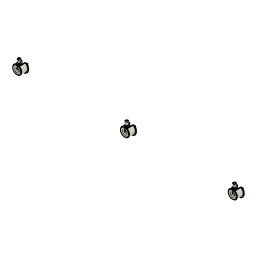
Rafix D20 Set (Autodesk Fusion 360 design; units mm, degrees)
description: Smart Rafix 20 Set
part number: Rafix 20 Set
description: Hafele Rafix S20 Connecting bolt
part number: Rafix S20 Bolt (263.20.xxx)
description: Hafele Rafix 20 Connector housing
part number: Rafix 20 (263.10.xxx)
Autodesk Fusion 360 part; units mm, degrees
sketch "Main Sketch" plane through (0, 0, 0) normal (0, 0, 1) x (1, 0, 0)
  line L0 (300, -10) -> (-300, -10)
  line L1 (-300, -10) -> (-300, 10)
  line L2 (-300, 10) -> (300, 10)
  line L3 (300, 10) -> (300, -10)
  line L4 (300, -10) -> (-300, 10) construction
  line L5 (-300, -10) -> (300, 10) construction
  circle A0 centre (-240, 0.5) radius 0.5
  circle A1 centre (240, 0.5) radius 0.5
  point P0 (-240, 0.5)
  point P1 (240, 0.5)
  dimension "d3" = 600
  dimension "d4" = 20
  dimension "d7" = 60
  dimension "d9" = 9.5
  dimension "d16" = 1
  dimension "d17" = 1
  dimension "d31" = 60
  constraint horizontal L0
  constraint perpendicular L0 L1
  constraint parallel L0 L2
  constraint parallel L1 L3
  constraint coincident L4 origin
  constraint coincident L5 origin
  constraint horizontal P0 P1
  constraint coincident P0 A0.centre
  constraint coincident P1 A1.centre
  measures "d3" distance of L0.start L0.end
  measures "d4" distance of L0 L2
  measures "d7" distance of L1 P0
  measures "d9" distance of L2 P0
  measures "d16" diameter of A0
  measures "d17" diameter of A1
  measures "d31" distance of L3 P1
extrude "Extrude3" add sketch "Main Sketch" along normal blind 10 contours A0 makes body 1
pattern_linear "R-Pattern1" count 3 spacing 240 along (1, 0, 0) of bodies 1 makes body 2 at (0.4994, 0.4751, 6.6667) makes body 3 at (240.0622, 0.0039, 3.3333)
ref_plane "WorkPlane1" through (-240, 0.5, 5) normal (-1, 0, 0) x (0, 0, 1)
sketch "Sketch2" plane through (-240, 0.5, 5) normal (-1, 0, 0) x (0, 1, 0)
  line L0 (0, 5) -> (0, -19.5056)
  line L1 (-1.5, 5) -> (-1.5, 3.5)
  line L2 (-1.5, 3.5) -> (-3, 3.5)
  line L3 (-3, 3.5) -> (-3, -6)
  line L4 (-10.5, 5) -> (9.5, 5)
  line L5 (-3, -6) -> (0, -6)
  line L6 (-1.5, 5) -> (-3.5, 5)
  line L7 (-3.5, 5) -> (-3.5, 8.5)
  line L8 (-3.5, 8.5) -> (-1.5, 8.5)
  line L9 (-1.5, 8.5) -> (-1.5, 11)
  line L10 (0, 14) -> (-3.5, 14)
  line L11 (-3.5, 14) -> (-3.5, 13.6)
  arc A0 (-3.5, 13.6) -> (-1.5, 11) centre (-0.81, 13.6) ccw
  line L12 (0, 5) -> (0, 14)
  point P0 (0, 5)
  point P1 (0, 5)
  dimension "d34" = 1.5
  dimension "d35" = 3
  dimension "d36" = 6
  dimension "d37" = 11
  dimension "d38" = 7
  dimension "d39" = 3.5
  dimension "d40" = 2.5
  dimension "d41" = 3
  dimension "d42" = 0.4
  dimension "d43" = 9
  dimension "d44" = 7
  constraint vertical L0
  constraint parallel L0 L1
  constraint perpendicular L1 L2
  constraint perpendicular L2 L3
  constraint coincident L1.start L4
  constraint coincident L0 L5.end
  constraint perpendicular L0 L5
  constraint coincident L4 L6.end
  constraint perpendicular L4 L7
  constraint perpendicular L1 L8
  constraint perpendicular L4 L9
  constraint horizontal L10
  constraint perpendicular L10 L11
  constraint coincident P0 L0.start
  constraint vertical L10.start P1
  constraint tangent L11 A0
  constraint coincident P1 P0
  measures "d34" distance of L2 L4
  measures "d37" distance of L3.end L4
  measures "d39" distance of L4 L8
  measures "d40" distance of L8.end L9.end
  measures "d42" distance of L10.end L11.end
  measures "d43" distance of L6.end L10
revolve "Revolve1" add sketch "Sketch2" angle 360 about axis through (-240, 0.5, 0) along (0, 0, 1) separate body makes body 4
chamfer "Chamfer1" distance 1.4 angle 45 2 edges at (-242.797, 1.5848, 1.5) (-242.797, 1.5848, 11) on bodies 4
fillet "Fillet1" radius 0.5 1 edges at (-243.2631, 1.7657, -3.5) on bodies 4
sketch "Sketch3" plane through (0, 0, -9) normal (0, 0, -1) x (1, 0, 0)
  circle A0 centre (-240, -0.5) radius 3.5
  line L0 (-243.8, 0.1) -> (-236.2, 0.1)
  line L1 (-236.2, 0.1) -> (-236.2, -1.1)
  line L2 (-236.2, -1.1) -> (-243.8, -1.1)
  line L3 (-243.8, -1.1) -> (-243.8, 0.1)
  line L4 (-243.8, 0.1) -> (-236.2, -1.1) construction
  line L5 (-236.2, 0.1) -> (-243.8, -1.1) construction
  line L6 (-240.6, 2.4) -> (-239.4, 2.4)
  line L7 (-239.4, 2.4) -> (-239.4, -3.4)
  line L8 (-239.4, -3.4) -> (-240.6, -3.4)
  line L9 (-240.6, -3.4) -> (-240.6, 2.4)
  line L10 (-240.6, 2.4) -> (-239.4, -3.4) construction
  line L11 (-239.4, 2.4) -> (-240.6, -3.4) construction
  circle A1 centre (-240, -0.5) radius 3.5
  point P0 (-240, -0.5)
  point P1 (-240, -0.5)
  point P2 (-240, -4)
  point P3 (-243.5, -0.5)
  dimension "d49" = 1.2
  dimension "d50" = 1.2
  dimension "d51" = 0.6
  dimension "d52" = 0.3
  constraint horizontal L0
  constraint perpendicular L0 L1
  constraint parallel L0 L2
  constraint parallel L1 L3
  constraint coincident L4 P1
  constraint coincident L5 P1
  constraint coincident P0 A0.centre
  constraint horizontal L6
  constraint perpendicular L6 L7
  constraint parallel L6 L8
  constraint parallel L7 L9
  constraint coincident L10 P1
  constraint coincident L11 P1
  constraint coincident P1 P0
  constraint coincident A1 P2
  constraint coincident A1 P3
  constraint vertical P1 P2
  constraint horizontal P1 P3
  measures "d49" distance of L0.end L1.end
  measures "d50" distance of L7.end L8.end
  measures "d51" distance of L8 P2
  measures "d52" distance of L3 P3
extrude "Extrude4" cut sketch "Sketch3" against normal blind 1.5 draft -10 contours A0 L0 L2 L7 A1 | A0 L0 L1 L2 A1 | A0 L0 L2 L9 A1 | A0 L0 L2 L3 A1 | L0 L2 L7 L9 | L0 L6 L7 L9 | L2 L7 L8 L9 bodies 4
thread "Thread1" "ISO Metric profile 6.0 M6x1 6g" major diameter 5.884 minor diameter 4.7435 pitch 1 angle 60 resizes the face on face at (-238.9739, 3.3191, 5.1333) on bodies 4
sketch "Sketch4" plane through (-240, 0.5, 5) normal (-1, 0, 0) x (0, 1, 0)
  line L0 (0, 10) -> (0, -10)
  line L1 (0, 5) -> (2.5, 5)
  line L2 (2.5, 5) -> (2.5, -8)
  line L3 (1.6, -6) -> (-1.6, -6)
  line L4 (0, -8) -> (2.5, -8)
  line L5 (3.5, 5) -> (-3.5, 5)
  dimension "d55" = 5
  dimension "d57" = 2
  constraint coincident L0 L1.start
  constraint perpendicular L0 L1
  constraint perpendicular L1 L2
  constraint coincident L0 L4.start
  constraint perpendicular L0 L4
  constraint collinear L1 L5
  measures "d57" distance of L3.start L4
copy_body "Body->Comp1" bodies 4 removing the originals makes body 5 in component "RafixBolt"
pattern_linear "00000000-0000-0000-0000-000000000000" [suppressed]
ref_plane "WorkPlane2" through (-240, 0.5, 5) normal (0, 1, 0) x (0, 0, 1)
ref_plane "WorkPlane3" through (-240, 10, 5) normal (0, 1, 0) x (0, 0, 1)
sketch "Sketch5" plane through (-240, 10, 5) normal (0, 1, 0) x (1, 0, 0)
  circle A0 centre (0, 14.5) radius 10
  line L0 (-4.7497, 5.7) -> (4.7497, 5.7)
  line L1 (3.5, 5) -> (-3.5, 5)
  dimension "d73" = 20
  dimension "d74" = 8.8
  dimension "d75" = 9.5
  constraint coincident A0 L0.start
  constraint coincident A0 L0.end
  constraint horizontal L0
  constraint vertical origin A0.centre
  measures "d73" diameter of A0
  measures "d74" distance of A0.centre L0
  measures "d75" distance of A0.centre L1
extrude "Extrude5" add sketch "Sketch5" against normal blind 14.2 separate body contours A0 L0 makes body 6
sketch "Sketch7" plane through (0, 10, 0) normal (0, 1, 0) x (-1, 0, 0)
  line L0 (244.7497, -0.7) -> (235.2503, -0.7)
  arc A0 (235.2503, -0.7) -> (244.7497, -0.7) centre (240, -9.5) ccw
  line L1 (250, -9.5) -> (230, -9.5)
  line L2 (230, -9.5) -> (230, -0.7)
  line L3 (230, -0.7) -> (250, -0.7)
  line L4 (250, -0.7) -> (250, -9.5)
  circle A1 centre (240, -9.5) radius 12
  dimension "d82" = 24
  constraint horizontal L1
  constraint vertical L2
  constraint horizontal L3
  constraint vertical L4
  constraint coincident A0.centre L1
  constraint tangent A0 L2
  constraint tangent A0 L4
  constraint collinear L0 L3
  constraint concentric A0 A1
  measures "d82" diameter of A1
extrude "Extrude7" add sketch "Sketch7" along normal blind 1.2 contours L0 A0 L1 L3 | A0 L3 L4 A1 | A0 L2 L3 A1 | A0 L2 L4 A1 | A0 L1 | L3 L4 A1 | L2 L3 A1 bodies 6
fillet "Fillet2" radius 2 2 edges at (-250, 10.6, -2.8668) (-230, 10.6, -2.8668) on bodies 6
fillet "Fillet3" radius 1 5 edges at (-230, 11.2, -1.4944) (-229.9272, 11.2, -2.8234) (-240, 11.2, -21.5) (-250.0728, 11.2, -2.8234) (-250, 11.2, -1.4944) on bodies 6
sketch "Sketch8" plane through (0, 0, -0.7) normal (0, 0, 1) x (-1, 0, 0)
  arc A0 (249, -11.2) -> (250, -10.2) centre (249, -10.2) ccw
  line L0 (250, -10.2) -> (250, -10)
  line L1 (250, -10) -> (244.7497, -10)
  line L2 (244.7497, -10) -> (244.7497, 4.2)
  line L3 (244.7497, 4.2) -> (235.2503, 4.2)
  line L4 (235.2503, 4.2) -> (235.2503, -10)
  line L5 (235.2503, -10) -> (230, -10)
  line L6 (230, -10) -> (230, -10.2)
  arc A1 (230, -10.2) -> (231, -11.2) centre (231, -10.2) ccw
  line L7 (231, -11.2) -> (249, -11.2)
  line L8 (236.2503, 3.2) -> (243.7497, 3.2)
  line L9 (243.7497, 3.2) -> (243.7497, -11.2)
  line L10 (243.7497, -11.2) -> (236.2503, -11.2)
  line L11 (236.2503, -11.2) -> (236.2503, 3.2)
  line L12 (236.2503, 3.2) -> (243.7497, -11.2) construction
  line L13 (243.7497, 3.2) -> (236.2503, -11.2) construction
  point P0 (240, -4)
  point P1 (240, 4.2)
  dimension "d89" = 1
  dimension "d91" = 1
  dimension "d92" = 7.4995
  constraint horizontal L8
  constraint perpendicular L8 L9
  constraint parallel L8 L10
  constraint parallel L9 L11
  constraint coincident L12 P0
  constraint coincident L13 P0
  constraint midpoint L3 P1
  constraint vertical P0 P1
  constraint collinear L7 L10
  measures "d89" distance of L2 L9
  measures "d91" distance of L3 L8
  measures "d92" distance of L9 L11
extrude "Extrude8" cut sketch "Sketch8" against normal blind 6.8 contours L7 L8 L9 L10 L11 bodies 6
fillet "Fillet4" radius 3.7495 2 edges at (-243.7497, -3.2, -4.1) (-236.2503, -3.2, -4.1) on bodies 6
ref_plane "WorkPlane4" through (-240, 10, -9.5) normal (0, 0, 1) x (1, 0, 0)
ref_plane "WorkPlane5" through (-240, 10, -10.5) normal (0, 0, 1) x (1, 0, 0)
ref_plane "WorkPlane6" through (-240, 10, 0) normal (0, 0, 1) x (1, 0, 0)
ref_plane "WorkPlane7" through (-240, 0.5, 5) normal (-1, 0, 0) x (0, 0, 1)
sketch "Sketch9" plane through (-240, 0.5, 5) normal (-1, 0, 0) x (0, 1, 0)
  line L0 (9.2, 15.5) -> (9.2, 10.5)
  line L1 (9.2, 10.5) -> (-3.5, 10.5)
  line L2 (-3.5, 10.5) -> (-3.5, 15.5)
  line L3 (10.7, 12.5) -> (10.7, 5.7)
  line L4 (-3.7, 12.5) -> (-3.7, 5.7)
  line L5 (23.9, 15.5) -> (-4.9, 15.5)
  point P0 (9.5, 14.5)
  dimension "d102" = 1.5
  dimension "d103" = 0.2
  dimension "d125" = 10
  constraint vertical L0
  constraint coincident L0.start L5
  constraint coincident L2.end L5
  measures "d102" distance of L0 L3
  measures "d103" distance of L2 L4
copy_body "Body->Comp3" bodies 6 removing the originals makes body 7 in component "Rafix 20"
sketch "Sketch1" plane through (-239.9998, 0.5495, 5) normal (-1, 0, 0) x (0, 1, 0) in component "Rafix 20"
  line L0 (23.9, 15.5) -> (-4.9, 15.5)
  line L1 (9.1505, 15.5) -> (-3.5495, 15.5)
  line L2 (-3.5495, 15.5) -> (-3.5495, 10.5)
  line L3 (-3.5495, 10.5) -> (9.1505, 10.5)
  line L4 (9.1505, 10.5) -> (9.1505, 15.5)
  line L5 (10.6505, 12.5) -> (10.6505, 5.7)
  line L6 (-3.7495, 12.5) -> (0, 12.5)
  line L7 (-3.7495, 12.5) -> (-3.7495, 5.7)
  line L8 (-3.7495, 5.7) -> (0, 5.7)
  line L9 (0, 5.7) -> (0, 12.5)
  dimension "d165" = 1.5
  dimension "d166" = 0.2
  dimension "d167" = 10
  constraint horizontal L1
  constraint vertical L2
  constraint horizontal L3
  constraint vertical L4
  constraint coincident L0 L1.start
  measures "d165" distance of L4 L5
  measures "d166" horizontal distance of L2.end L6.start
revolve "Revolve1'" cut sketch "Sketch1" angle 360 about axis through (-239.9998, 24.4495, -10.5) along (0, -1, 0) contours L0 L1 L2 L3 L4 L6 L9 | L2 L3 L6 L9 bodies 7 in component "Rafix 20"
sketch "Sketch2 (2)" plane through (-239.9998, 0.5495, 5) normal (-1, 0, 0) x (0, 1, 0) in component "Rafix 20"
  line L0 (6.2505, 10.4) -> (-3.7495, 10.4)
  line L1 (-3.7495, 10.4) -> (-3.7495, 8.9)
  line L2 (-3.7495, 8.9) -> (6.2505, 8.9)
  line L3 (6.2505, 8.9) -> (6.2505, 10.4)
  spline S0 degree 3 poles (0, 12.1922) (-0.2518, 12.1922) (-0.5045, 12.1626) (-0.9967, 12.0537) (-1.2363, 11.9749) (-1.9185, 11.6988) (-2.3257, 11.4645) (-2.9701, 11.0614) (-3.2564, 10.8602) (-3.4872, 10.6937) (-3.5199, 10.6698) (-3.5495, 10.6482) knots 0 0 0 0 0.07553 0.07553 0.15106 0.15106 0.302121 0.302121 0.450006 0.450006 0.477033 0.477033 0.477033 0.477033
  line L4 (-3.5495, 10.6482) -> (-3.5495, 12.5)
  line L5 (-3.7495, 12.5) -> (-3.5495, 12.5)
  line L6 (-3.7495, 12.5) -> (-3.7495, 5.7)
  line L7 (-3.7495, 5.7) -> (0, 5.7)
  line L8 (0, 5.7) -> (0, 12.1922)
  line L9 (10.6505, 5.7) -> (0, 5.7)
  dimension "d170" = 1.5
  dimension "d171" = 3.2
  dimension "d172" = 10
  constraint horizontal L0
  constraint vertical L1
  constraint horizontal L2
  constraint vertical L3
  constraint collinear L1 L6
  measures "d170" distance of L0.start L2.end
  measures "d171" distance of L2 L9
  measures "d172" distance of L1.end L3
extrude "Extrude1" add sketch "Sketch2 (2)" along normal up to surface (3.75 mm away) and the other way up to surface (3.7495 mm away) contours L0 L2 L3 L8 | L0 L1 L2 L6 L8 bodies 7 in component "Rafix 20"
sketch "Sketch3 (2)" plane through (0, 0, -3.9) normal (0, 0, 1) x (-1, 0, 0) in component "Rafix 20"
  arc A0 (239.9998, 3.2) -> (236.2503, -0.5495) centre (239.9998, -0.5495) ccw
  line L0 (236.2503, -0.5495) -> (236.2503, -6.8)
  line L1 (236.2503, -6.8) -> (243.7497, -6.8)
  line L2 (243.7497, -6.8) -> (243.7497, -0.5495)
  arc A1 (243.7497, -0.5495) -> (240.0002, 3.2) centre (240.0002, -0.5495) ccw
  line L3 (240.0002, 3.2) -> (239.9998, 3.2)
  line L4 (243.7497, -6.8) -> (242.5497, -3.8)
  line L5 (236.2503, -6.8) -> (237.4503, -3.8)
  circle A2 centre (239.9998, -0.5495) radius 1.5
  circle A3 centre (239.9998, -0.5495) radius 2.55
  line L6 (242.5497, -3.8) -> (237.4503, -3.8)
  line L7 (242.5497, -3.8) -> (242.5497, -0.5495)
  line L8 (237.4503, -3.8) -> (237.4503, -0.5004)
  dimension "d178" = 3
  dimension "d217" = 1.2
  dimension "d218" = 1.2
  constraint coincident L1.end L2.start
  constraint coincident L0.end L1.start
  constraint horizontal L4.end L5.end
  constraint concentric A2 A3
  constraint perpendicular L6 L7
  constraint perpendicular L6 L8
  constraint tangent A3 L7
  constraint coincident A3 L7.end
  constraint coincident A3 L8.end
  measures "d178" vertical distance of L1.end L4.end
  measures "d217" horizontal distance of L1.end L4.end
  measures "d218" horizontal distance of L0.end L5.end
extrude "Extrude2" cut sketch "Sketch3 (2)" against normal up to surface (1.5 mm away) contours A3 | L1 L4 L5 L6 | A3 L6 L7 L8 | A2 bodies 7 in component "Rafix 20"
sketch "Sketch4 (2)" plane through (0, 11.2, 0) normal (0, 1, 0) x (-1, 0, 0) in component "Rafix 20"
  line L0 (243.7497, -0.7) -> (243.7497, -7.5)
  line L1 (243.7497, -7.5) -> (236.2503, -7.5)
  line L2 (236.2503, -7.5) -> (236.2503, -0.7)
  line L3 (236.2503, -0.7) -> (231, -0.7)
  line L4 (231, -0.7) -> (231, -2.2889)
  arc A0 (230.5714, -3.8341) -> (231, -2.2889) centre (228, -2.2889) ccw
  arc A1 (230.5714, -3.8341) -> (249.4286, -3.8341) centre (240, -9.5) ccw
  arc A2 (249, -2.2889) -> (249.4286, -3.8341) centre (252, -2.2889) ccw
  line L5 (249, -2.2889) -> (249, -0.7)
  line L6 (249, -0.7) -> (243.7497, -0.7)
  line L7 (243.7497, -9.5) -> (236.2503, -9.5) construction
  line L8 (236.2503, -9.5) -> (236.2503, -16.5)
  line L9 (236.2503, -16.5) -> (243.7497, -16.5) construction
  line L10 (243.7497, -16.5) -> (243.7497, -9.5)
  line L11 (243.7497, -9.5) -> (236.2503, -16.5) construction
  line L12 (236.2503, -9.5) -> (243.7497, -16.5) construction
  arc A3 (236.2503, -16.5) -> (243.7497, -16.5) centre (240, -7.2296) ccw
  arc A4 (243.7497, -9.5) -> (236.2503, -9.5) centre (240, -18.7704) ccw
  point P0 (240, -13)
  dimension "d181" = 7
  dimension "d182" = 2
  dimension "d183" = 10
  dimension "d184" = 10
  constraint horizontal L7
  constraint perpendicular L7 L8
  constraint parallel L7 L9
  constraint parallel L8 L10
  constraint coincident L11 P0
  constraint coincident L12 P0
  constraint collinear L2 L8
  constraint collinear L0 L10
  measures "d181" distance of L7 L9
  measures "d182" distance of L1 L7
  measures "d183" radius of A3
  measures "d184" radius of A4
extrude "Extrude3'" cut sketch "Sketch4 (2)" against normal blind 1.5 contours L8 L10 A3 A4 bodies 7 in component "Rafix 20"
fillet "Fillet1'" radius 2 4 edges at (-236.2503, 10.45, -16.5) (-243.7497, 10.45, -16.5) (-243.7497, 10.45, -9.5) (-236.2503, 10.45, -9.5) on bodies 7 in component "Rafix 20"
revolve "Revolve2" add sketch "Sketch1" angle 360 about axis through (-239.9998, 24.4495, -10.5) along (0, -1, 0) separate body contours L0 L1 L2 L3 L4 L6 L9 | L2 L3 L6 L9 makes body 8 in component "Rafix 20"
sketch "Sketch5 (2)" plane through (0, 9.7, 0) normal (0, 1, 0) x (-1, 0, 0) in component "Rafix 20"
  circle A0 centre (239.9998, -10.5) radius 5
  line L0 (235.9998, -9.9) -> (243.9998, -9.9)
  line L1 (243.9998, -9.9) -> (243.9998, -11.1)
  line L2 (243.9998, -11.1) -> (235.9998, -11.1)
  line L3 (235.9998, -11.1) -> (235.9998, -9.9)
  line L4 (235.9998, -9.9) -> (243.9998, -11.1) construction
  line L5 (243.9998, -9.9) -> (235.9998, -11.1) construction
  line L6 (239.3998, -6.5) -> (240.5998, -6.5)
  line L7 (240.5998, -6.5) -> (240.5998, -14.5)
  line L8 (240.5998, -14.5) -> (239.3998, -14.5)
  line L9 (239.3998, -14.5) -> (239.3998, -6.5)
  line L10 (239.3998, -6.5) -> (240.5998, -14.5) construction
  line L11 (240.5998, -6.5) -> (239.3998, -14.5) construction
  point P0 (239.9998, -10.5)
  point P1 (239.9998, -10.5)
  dimension "d191" = 8
  dimension "d192" = 1.2
  dimension "d193" = 1.2
  dimension "d194" = 8
  constraint horizontal L0
  constraint perpendicular L0 L1
  constraint parallel L0 L2
  constraint parallel L1 L3
  constraint coincident L4 P1
  constraint coincident L5 P1
  constraint coincident P0 A0.centre
  constraint horizontal L6
  constraint perpendicular L6 L7
  constraint parallel L6 L8
  constraint parallel L7 L9
  constraint coincident L10 P1
  constraint coincident L11 P1
  constraint coincident P1 P0
  measures "d191" distance of L1.end L2.end
  measures "d192" distance of L0.end L1.end
  measures "d193" distance of L7.end L8.end
  measures "d194" distance of L6.end L7.end
extrude "Extrude4'" cut sketch "Sketch5 (2)" against normal blind 2 draft -5 contours L0 L2 L3 L9 | L0 L6 L7 L9 | L0 L2 L7 L9 | L0 L1 L2 L7 | L2 L7 L8 L9 bodies 8 in component "Rafix 20"
sketch "Sketch6" plane through (-239.9998, 0.5495, 5) normal (-1, 0, 0) x (0, 1, 0) in component "Rafix 20"
  line L0 (23.9, 15.5) -> (-4.9, 15.5)
  line L1 (6.5505, 15.5) -> (-3.4495, 15.5)
  line L2 (-3.4495, 15.5) -> (-3.4495, 11.6425)
  line L3 (-3.4495, 11.6425) -> (6.5505, 11.6425)
  line L4 (6.5505, 11.6425) -> (6.5505, 15.5)
  line L5 (7.1505, 15.075) -> (7.1505, 15.925)
  line L6 (-3.5495, 10.6482) -> (-3.5495, 12.5)
  line L7 (-0.0495, 10.4) -> (-0.0495, 11.6425) construction
  line L8 (9.4505, 8.3191) -> (9.4505, 26.5) construction
  line L9 (9.1505, 20.5) -> (9.1505, 10.5)
  line L10 (-3.5495, 20.5) -> (-3.5495, 10.5)
  line L11 (-2.4495, 10.4) -> (2.3505, 10.4)
  line L12 (2.3505, 10.4) -> (2.3505, 11.6425)
  line L13 (2.3505, 11.6425) -> (-2.4495, 11.6425)
  line L14 (-2.4495, 11.6425) -> (-2.4495, 10.4)
  line L15 (-2.4495, 10.4) -> (2.3505, 11.6425) construction
  line L16 (2.3505, 10.4) -> (-2.4495, 11.6425) construction
  line L17 (3.2505, 10.4) -> (0, 10.4)
  point P0 (-0.0495, 11.0213)
  dimension "d197" = 0.6
  dimension "d198" = 0.1
  dimension "d199" = 7.715
  dimension "d200" = 9.5
  dimension "d201" = 4.8
  constraint horizontal L1
  constraint vertical L2
  constraint horizontal L3
  constraint vertical L4
  constraint coincident L0 L1.start
  constraint vertical L7
  constraint coincident L3 L7.end
  constraint horizontal L11
  constraint perpendicular L11 L12
  constraint parallel L11 L13
  constraint parallel L12 L14
  constraint coincident L15 P0
  constraint coincident L16 P0
  constraint midpoint L7 P0
  constraint collinear L3 L13
  constraint coincident L11 L17.end
  measures "d197" distance of L4 L5
  measures "d198" distance of L2.end L6
  measures "d200" distance of L7.end L8
  measures "d201" distance of L12.end L13.end
revolve "Revolve3" cut sketch "Sketch6" angle 90 about axis through (-239.9998, 24.4495, -10.5) along (0, -1, 0) second angle 90 bodies 7 8 in component "Rafix 20"
sketch "Sketch7 (2)" plane through (0, -4.2, 0) normal (0, -1, 0) x (1, 0, 0) in component "Rafix 20"
  arc A0 (-244.7497, -0.7) -> (-235.2503, -0.7) centre (-240, -9.5) ccw
  circle A1 centre (-240, -9.5) radius 10
  line L0 (-243.1225, 0) -> (-236.8775, 0)
  dimension "d212" = 20
  dimension "d213" = 9.5
  constraint concentric A0 A1
  constraint coincident A1 L0.start
  constraint coincident A1 L0.end
  constraint horizontal L0
  measures "d212" diameter of A1
  measures "d213" distance of A0.centre L0
extrude "Extrude5'" add sketch "Sketch7 (2)" against normal blind 14.3 separate body contours A0 A1 L0 makes body 9 in component "Rafix 20"
chamfer "Chamfer1'" distance 1 angle 45 1 edges at (-240, -4.2, -19.5) on bodies 7 in component "Rafix 20"
pattern_linear "00000000-0000-0000-0000-000000000000'" [suppressed]
sketch "Sketch1 (2)" plane through (0, 0, 0) normal (0, 0, 1) x (1, 0, 0) in component "RafixBolt"
  circle A0 centre (-240, 0.5) radius 2.5
  circle A1 centre (-240, 0.5) radius 3.5
  dimension "d214" = 5
  constraint coincident A0.centre A1.centre
  measures "d214" diameter of A0
extrude "Extrude2'" add sketch "Sketch1 (2)" along normal blind 13 separate body contours A0 makes body 10 in component "RafixBolt"
component "RafixBolt" placed x (1, 0, 0) y (0, 1, 0) z (0, 0, 1) at (0, 0, 0)
component "RafixBolt" placed x (1, 0, 0) y (0, 1, 0) z (0, 0, 1) at (240, 0, 0)
component "RafixBolt" placed x (1, 0, 0) y (0, 1, 0) z (0, 0, 1) at (480, 0, 0)
component "Rafix 20" placed x (1, 0, 0) y (0, 1, 0) z (0, 0, 1) at (-0.0002, -0.0495, 0)
component "Rafix 20" placed x (1, 0, 0) y (0, 1, 0) z (0, 0, 1) at (239.9998, -0.0495, 0)
component "Rafix 20" placed x (1, 0, 0) y (0, 1, 0) z (0, 0, 1) at (479.9998, -0.0495, 0)
hidden bodies 1 2 3 10 9
equation "ContactPatchLength = 600 mm"
equation "ContactPatchWidth = 20 mm"
equation "d3 = ContactPatchLength"
equation "d4 = ContactPatchWidth"
equation "Offset1 = if(( ContactPatchLength - UserOffset1 - UserOffset2 ) >= MinDistance; UserOffset1; ContactPatchLength / 2)"
equation "Offset2 = if(( ContactPatchLength - UserOffset1 - UserOffset2 ) >= MinDistance; UserOffset2; Offset1)"
equation "d7 = Offset1"
equation "d9 = Coord_Y"
equation "Coord_Y = DimA"
equation "PlacingLength = ContactPatchLength - Offset1 - Offset2"
equation "NumberOfIntervals = ceil(PlacingLength / MaxDistance)"
equation "MaxDistance = 300 mm" comment "Max distance between components"
equation "NumberOfComponents = if(PlacingLength >= MinDistance; NumberOfIntervals + 1; 1)"
equation "SpaceBetween = if(PlacingLength >= MinDistance; PlacingLength / NumberOfIntervals; 0 mm)"
equation "d24 = NumberOfComponents"
equation "d26 = -SpaceBetween"
equation "MinDistance = 32 mm" comment "Min distance between components"
equation "UserOffset1 = 60 mm" comment "Distance from the Edge"
equation "UserOffset2 = 60 mm" comment "Distance from the Edge"
equation "d31 = Offset2"
equation "RafixBoltLength = ( if(NestledBoardT <= 16 mm; 11; 15) ) * 1 mm" comment "Rafix Bolt Length L=11 if Nestled Board Thickness <=16 or L=15 if Thickness >16"
equation "d37 = RafixBoltLength"
equation "d50 = d49"
equation "d63 = NumberOfComponents"
equation "d65 = -SpaceBetween"
equation "PillarBoardT = 18 mm" comment "System Automatically maps this parameter with the board"
equation "NestledBoardT = 16 mm" comment "System Automatically maps this parameter with the boardSystem Automatically maps this parameter with the board"
equation "DimA = ( if(PillarBoardT <= 16 mm; 8; 9.5) ) * 1 mm" comment "Dimension for Rafix thickness control. If Pillar Board Thickness <=16 mm, then Dim A = 8, otherwise - 9.5"
equation "d72 = DimA"
equation "DrillingDepth = ( if(PillarBoardT <= 16 mm; 12.7; 14.2) ) * 1 mm" comment "Parameter controls Rafix thickness according to the pillar board T. If Thickness is <=16, than Drilling Depth =12.7; otherwise 14.2"
equation "d77 = -DrillingDepth"
equation "d93 = -d74 + 2 mm"
equation "d96 = ( 7.499 / 2 ) * 1 mm"
equation "d184 = d183"
equation "d200 = DimA"
equation "d204 = -DrillingDepth - 0.1 mm"
equation "d207 = NumberOfComponents"
equation "d209 = SpaceBetween"
equation "d215 = RafixBoltLength + 2 mm"
named bodies: "RafixBolt", "Rafix 20", "Cam", "Rafix Hole", "Bolt Hole"
